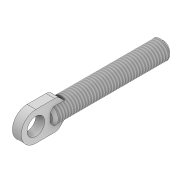
# Autodesk Inventor part: FRC220-1S
Saved by Autodesk Inventor 2020 (Build 240168000, 168)
## iProperties
Created: 2020-02-19
Part Number: FRC220-1S
Material: Generic
Document SubType Name: Modeling
Designer: Juan Carlos Botero
Density: 1 g/cm^3
Appearance: Default
Mass: 11.7915 g
Surface Area: 50.179 cm^2
Volume: 11.7915 cm^3
Author: Juan Carlos Botero
Title: SOPORTE MOVIL
Autodesk Inventor part; units mm, degrees
ref_plane "YZ Plane" through (0, 0, 0) normal (1, 0, 0) x (0, 1, 0)
ref_plane "XZ Plane" through (0, 0, 0) normal (0, 1, 0) x (-1, 0, 0)
ref_plane "XY Plane" through (0, 0, 0) normal (0, 0, 1) x (1, 0, 0)
sketch "Sketch1" plane through (0, 0, 0) normal (0, 0, 1) x (1, 0, 0)
  circle A0 centre (0, 0) radius 6.35
  dimension "d0" = 12.7
  constraints: 1 centre point, 1 coincident
  measures "d0" diameter of A0
extrude "Extrusion1" add sketch "Sketch1" along normal mid plane 80
sketch "Sketch2" plane through (0, 0, 40) normal (0, 0, 1) x (1, 0, 0)
  line L0 (-3, -13.1035) -> (3, -13.1035)
  line L1 (3, -13.1035) -> (3, 13.1035)
  line L2 (3, 13.1035) -> (-3, 13.1035)
  line L3 (-3, 13.1035) -> (-3, -13.1035)
  line L4 (-3, -13.1035) -> (3, 13.1035) construction
  line L5 (3, -13.1035) -> (-3, 13.1035) construction
  point P0 (0, 0)
  dimension "d3" = 6
  constraints: 12 end point, 2 midpoint, 2 parallel, 1 horizontal, 1 perpendicular
  measures "d3" distance of L2.end L1.end
extrude "Extrusion2" cut sketch "Sketch2" against normal blind 10
sketch "Sketch3" plane through (0, 0, 30) normal (0, 0, 1) x (1, 0, 0)
  line L0 (-3, -10) -> (3, -10)
  line L1 (3, -10) -> (3, 10)
  line L2 (3, 10) -> (-3, 10)
  line L3 (-3, 10) -> (-3, -10)
  line L4 (-3, -10) -> (3, 10) construction
  line L5 (3, -10) -> (-3, 10) construction
  point P0 (0, 0)
  dimension "d6" = 6
  dimension "d7" = 20
  constraints: 12 end point, 2 midpoint, 2 parallel, 1 horizontal, 1 perpendicular
  measures "d6" distance of L2.end L1.end
  measures "d7" distance of L1.end L0.end
extrude "Extrusion3" add sketch "Sketch3" along normal blind 30 separate body
fillet "Fillet1" radius 10 2 edges at (0, 10, 60) (0, -10, 60)
thread "Thread1" size "1/2-13 UNC" class "2A" standard "ANSI Unified Screw Threads" full length
chamfer "Chamfer1" distance 2 angle 45 1 edges at (-6.35, 0, -40)
sketch "Sketch5" plane through (-3, -10, 30) normal (-1, 0, 0) x (0, 0, 1)
  arc A0 (20, 0) -> (20, 20) centre (20, 10) ccw projected
  line L0 (0, 20) -> (20, 20) projected
  line L1 (0, 20) -> (0, 0) projected
  line L2 (0, 0) -> (20, 0) projected
  circle A1 centre (20, 10) radius 6
  point P0 (-30, 10)
  dimension "d20" = 12
  constraints: 1 centre point, 1 coincident
  measures "d20" diameter of A1
extrude "Extrusion5" cut sketch "Sketch5" against normal through all contours A1 bodies 2
chamfer "Chamfer2" distance 2 angle 45 3 edges at (-6.35, 0, 40) (5.4485, -3.2613, 40) (5.4485, 3.2613, 40)
chamfer "Chamfer3" distance 5 angle 45 2 edges at (0, -10, 30) (0, 10, 30)
fillet "Fillet2" radius 5 2 edges at (0, -10, 35) (0, 10, 35)
body "Solid1"
body "Solid2"
